Autodesk Fusion 360 part; units mm, degrees
(part 2 of 2)
sketch "Sketch3" plane through (0, 0, 0) normal (0, 0, 1) x (1, 0, 0)
  line L0 (-10.0312, 59.3426) -> (-10.0312, 45.3434)
  line L1 (-24.0307, 45.3434) -> (-24.0307, 59.3426)
  line L2 (-24.0307, 26.2934) -> (-24.0307, 40.2927)
  line L3 (-10.0312, 40.2927) -> (-10.0312, 26.2934)
  line L4 (-24.0307, 7.2434) -> (-24.0307, 21.2427)
  line L5 (-10.0312, 7.2434) -> (-24.0307, 7.2434)
  line L6 (-10.0312, 21.2427) -> (-10.0312, 7.2434)
  line L7 (-24.0307, -11.8066) -> (-24.0307, 2.1927)
  line L8 (-10.0312, -11.8066) -> (-24.0307, -11.8066)
  line L9 (-10.0312, 2.1927) -> (-10.0312, -11.8066)
  line L10 (-24.0307, -30.8568) -> (-24.0307, -16.8574)
  line L11 (-10.0312, -30.8568) -> (-24.0307, -30.8568)
  line L12 (-10.0312, -16.8574) -> (-10.0312, -30.8568)
  line L13 (-4.9807, 26.2934) -> (-4.9807, 40.2927)
  line L14 (9.0186, 26.2934) -> (-4.9807, 26.2934)
  line L15 (9.0186, 40.2927) -> (9.0186, 26.2934)
  line L16 (-4.9807, 7.2434) -> (-4.9807, 21.2427)
  line L17 (9.0186, 7.2434) -> (-4.9807, 7.2434)
  line L18 (9.0186, 21.2427) -> (9.0186, 7.2434)
  line L19 (-4.9807, -11.8066) -> (-4.9807, 2.1927)
  line L20 (9.0186, -11.8066) -> (-4.9807, -11.8066)
  line L21 (9.0186, 2.1927) -> (9.0186, -11.8066)
  line L22 (-4.9807, -30.8568) -> (-4.9807, -16.8574)
  line L23 (9.0186, -30.8568) -> (-4.9807, -30.8568)
  line L24 (9.0186, -16.8574) -> (9.0186, -30.8568)
  line L25 (14.0693, 26.2934) -> (14.0693, 40.2927)
  line L26 (28.0686, 26.2934) -> (14.0693, 26.2934)
  line L27 (14.0693, 40.2927) -> (28.0686, 40.2927)
  line L28 (14.0693, 7.2434) -> (14.0693, 21.2427)
  line L29 (28.0686, 7.2434) -> (14.0693, 7.2434)
  line L30 (28.0686, 21.2427) -> (28.0686, 7.2434)
  line L31 (14.0693, -11.8066) -> (14.0693, 2.1927)
  line L32 (28.0686, -11.8066) -> (14.0693, -11.8066)
  line L33 (28.0686, 2.1927) -> (28.0686, -11.8066)
  line L34 (14.0693, -30.8568) -> (14.0693, -16.8574)
  line L35 (28.0686, -30.8568) -> (14.0693, -30.8568)
  line L36 (28.0686, -16.8574) -> (28.0686, -30.8568)
  line L37 (33.1193, 26.2934) -> (33.1193, 40.2927)
  line L38 (47.1186, 26.2934) -> (33.1193, 26.2934)
  line L39 (47.1186, 40.2927) -> (47.1186, 26.2934)
  line L40 (33.1193, 45.3434) -> (33.1193, 59.3426)
  line L41 (39.6196, 19.9928) -> (33.3493, 19.9928)
  line L42 (32.1492, 18.2691) -> (32.1492, 14.9685)
  line L43 (32.1492, 14.9685) -> (33.3493, 14.9685)
  line L44 (33.3493, 13.2431) -> (37.8197, 13.2431)
  line L45 (33.3493, 14.9685) -> (33.3493, 13.2431)
  line L46 (33.3493, 18.2691) -> (32.1492, 18.2691)
  line L47 (33.3493, 19.9928) -> (33.3493, 18.2691)
  line L48 (37.8197, 13.2431) -> (37.8197, 11.7177)
  line L49 (37.8197, 11.7177) -> (33.1193, 11.7177)
  line L50 (42.4196, 13.2431) -> (45.6496, 13.2431)
  line L51 (47.1186, -2.2816) -> (47.1186, 11.7177)
  line L52 (47.1186, 11.7177) -> (42.4196, 11.7177)
  line L53 (42.4196, -2.2816) -> (47.1186, -2.2816)
  line L54 (33.1193, -2.2816) -> (37.8197, -2.2816)
  line L55 (33.1193, 11.7177) -> (33.1193, -2.2816)
  line L56 (37.8197, -3.8074) -> (33.3493, -3.8074)
  line L57 (32.1492, -5.5325) -> (32.1492, -8.8317)
  line L58 (33.3493, -10.5567) -> (39.6196, -10.5567)
  line L59 (45.6496, -10.5567) -> (45.6496, -3.8074)
  line L60 (42.4196, -10.5567) -> (45.6496, -10.5567)
  line L61 (45.6496, -3.8074) -> (42.4196, -3.8074)
  line L62 (39.6196, -11.3822) -> (42.4196, -11.3822)
  line L63 (42.4196, 20.8183) -> (39.6196, 20.8183)
  line L64 (45.6496, 13.2431) -> (45.6496, 19.9928)
  line L65 (45.6496, 19.9928) -> (42.4196, 19.9928)
  line L66 (42.4196, 19.9928) -> (42.4196, 20.8183)
  line L67 (39.6196, 20.8183) -> (39.6196, 19.9928)
  line L68 (42.4196, 11.7177) -> (42.4196, 13.2431)
  line L69 (37.8197, -2.2816) -> (37.8197, -3.8074)
  line L70 (42.4196, -3.8074) -> (42.4196, -2.2816)
  line L71 (33.3493, -5.5325) -> (32.1492, -5.5325)
  line L72 (33.3493, -3.8074) -> (33.3493, -5.5325)
  line L73 (32.1492, -8.8317) -> (33.3493, -8.8317)
  line L74 (33.3493, -8.8317) -> (33.3493, -10.5567)
  line L75 (39.6196, -10.5567) -> (39.6196, -11.3822)
  line L76 (42.4196, -11.3822) -> (42.4196, -10.5567)
  line L77 (14.0693, -49.9068) -> (14.0693, -35.9059)
  line L78 (28.0686, -49.9068) -> (14.0693, -49.9068)
  line L79 (28.0686, -35.9059) -> (28.0686, -49.9068)
  line L80 (33.1193, -26.3823) -> (33.1193, -40.3818)
  line L81 (47.1186, -40.3818) -> (47.1186, -26.3823)
  line L82 (45.6496, -48.6569) -> (45.6496, -41.9073)
  line L83 (45.6496, -24.8568) -> (45.6496, -18.1071)
  line L84 (47.1186, -26.3823) -> (42.4196, -26.3823)
  line L85 (37.8197, -26.3823) -> (33.1193, -26.3823)
  line L86 (33.1193, -40.3818) -> (37.8197, -40.3818)
  line L87 (42.4196, -40.3818) -> (47.1186, -40.3818)
  line L88 (45.6496, -41.9073) -> (42.4196, -41.9073)
  line L89 (37.8197, -41.9073) -> (33.3493, -41.9073)
  line L90 (33.3493, -48.6569) -> (39.6196, -48.6569)
  line L91 (39.6196, -49.4824) -> (42.4196, -49.4824)
  line L92 (42.4196, -48.6569) -> (45.6496, -48.6569)
  line L93 (32.1492, -43.6326) -> (32.1492, -46.9316)
  line L94 (33.3493, -24.8568) -> (37.8197, -24.8568)
  line L95 (42.4196, -24.8568) -> (45.6496, -24.8568)
  line L96 (45.6496, -18.1071) -> (42.4196, -18.1071)
  line L97 (39.6196, -18.1071) -> (33.3493, -18.1071)
  line L98 (42.4196, -17.2817) -> (39.6196, -17.2817)
  line L99 (32.1492, -19.8325) -> (32.1492, -23.1315)
  line L100 (42.4196, -26.3823) -> (42.4196, -24.8568)
  line L101 (37.8197, -24.8568) -> (37.8197, -26.3823)
  line L102 (32.1492, -23.1315) -> (33.3493, -23.1315)
  line L103 (33.3493, -23.1315) -> (33.3493, -24.8568)
  line L104 (33.3493, -19.8325) -> (32.1492, -19.8325)
  line L105 (33.3493, -18.1071) -> (33.3493, -19.8325)
  line L106 (39.6196, -17.2817) -> (39.6196, -18.1071)
  line L107 (42.4196, -18.1071) -> (42.4196, -17.2817)
  line L108 (37.8197, -40.3818) -> (37.8197, -41.9073)
  line L109 (42.4196, -41.9073) -> (42.4196, -40.3818)
  line L110 (32.1492, -46.9316) -> (33.3493, -46.9316)
  line L111 (33.3493, -46.9316) -> (33.3493, -48.6569)
  line L112 (33.3493, -43.6326) -> (32.1492, -43.6326)
  line L113 (33.3493, -41.9073) -> (33.3493, -43.6326)
  line L114 (39.6196, -48.6569) -> (39.6196, -49.4824)
  line L115 (42.4196, -49.4824) -> (42.4196, -48.6569)
  line L116 (-0.5063, -35.9059) -> (-14.5057, -35.9059)
  line L117 (-16.0312, -37.3762) -> (-22.7808, -37.3762)
  line L118 (-23.6063, -40.6078) -> (-23.6063, -43.4066)
  line L119 (-14.5057, -49.9068) -> (-0.5063, -49.9068)
  line L120 (-21.0555, -50.8756) -> (-17.7565, -50.8756)
  line L121 (-22.7808, -43.4066) -> (-22.7808, -49.6767)
  line L122 (-22.7808, -37.3762) -> (-22.7808, -40.6078)
  line L123 (-14.5057, -35.9059) -> (-14.5057, -40.6078)
  line L124 (-14.5057, -45.2063) -> (-14.5057, -49.9068)
  line L125 (-16.0312, -49.6767) -> (-16.0312, -45.2063)
  line L126 (7.7689, -37.3762) -> (1.0192, -37.3762)
  line L127 (7.7689, -49.6767) -> (7.7689, -43.4066)
  line L128 (7.7689, -40.6078) -> (7.7689, -37.3762)
  line L129 (1.0192, -45.2063) -> (1.0192, -49.6767)
  line L130 (2.7445, -50.8756) -> (6.0436, -50.8756)
  line L131 (-0.5063, -45.2063) -> (1.0192, -45.2063)
  line L132 (-0.5063, -49.9068) -> (-0.5063, -45.2063)
  line L133 (-17.7565, -49.6767) -> (-16.0312, -49.6767)
  line L134 (-22.7808, -49.6767) -> (-21.0555, -49.6767)
  line L135 (-16.0312, -40.6078) -> (-16.0312, -37.3762)
  line L136 (-0.5063, -40.6078) -> (-0.5063, -35.9059)
  line L137 (1.0192, -40.6078) -> (-0.5063, -40.6078)
  line L138 (1.0192, -37.3762) -> (1.0192, -40.6078)
  line L139 (8.5943, -43.4066) -> (8.5943, -40.6078)
  line L140 (8.5943, -40.6078) -> (7.7689, -40.6078)
  line L141 (7.7689, -43.4066) -> (8.5943, -43.4066)
  line L142 (1.0192, -49.6767) -> (2.7445, -49.6767)
  line L143 (2.7445, -49.6767) -> (2.7445, -50.8756)
  line L144 (6.0436, -50.8756) -> (6.0436, -49.6767)
  line L145 (6.0436, -49.6767) -> (7.7689, -49.6767)
  line L146 (-21.0555, -49.6767) -> (-21.0555, -50.8756)
  line L147 (-17.7565, -50.8756) -> (-17.7565, -49.6767)
  line L148 (-14.5057, -40.6078) -> (-16.0312, -40.6078)
  line L149 (-16.0312, -45.2063) -> (-14.5057, -45.2063)
  line L150 (-22.7808, -40.6078) -> (-23.6063, -40.6078)
  line L151 (-23.6063, -43.4066) -> (-22.7808, -43.4066)
  line L152 (-30.0717, 77.1478) -> (79.9283, 77.1478)
  line L153 (-30.0717, -55.8522) -> (-30.0717, 77.1478)
  line L154 (79.9283, -55.8522) -> (-30.0717, -55.8522)
  line L155 (79.9283, -55.8522) -> (79.9283, 77.1478)
  line L156 (0.5583, 54.6978) -> (21.2983, 54.6978)
  line L157 (21.2983, 54.6978) -> (21.2983, 64.5578)
  line L158 (0.5583, 64.5578) -> (0.5583, 54.6978)
  line L159 (86.9283, -55.8522) -> (86.9283, 77.1478)
  line L160 (-30.0717, 84.1478) -> (79.9283, 84.1478)
  line L161 (-37.0717, -55.8522) -> (-37.0717, 77.1478)
  line L162 (79.9283, -62.8522) -> (-30.0717, -62.8522)
  arc A0 (-30.0717, 84.1478) -> (-37.0717, 77.1478) centre (-30.0717, 77.1478) ccw
  arc A1 (86.9283, 77.1478) -> (79.9283, 84.1478) centre (79.9283, 77.1478) ccw
  arc A2 (79.9283, -62.8522) -> (86.9283, -55.8522) centre (79.9283, -55.8522) ccw
  arc A3 (-37.0717, -55.8522) -> (-30.0717, -62.8522) centre (-30.0717, -55.8522) ccw
  line L163 (-24.7, 58.6) -> (-11, 58.6)
  line L164 (-11, 58.6) -> (-11, 44.5)
  line L165 (-11, 44.5) -> (-24.7, 44.5)
  line L166 (-24.7, 44.5) -> (-24.7, 58.6)
  line L167 (34.1862, 59.1014) -> (48.2214, 59.1014)
  line L168 (48.2214, 59.1014) -> (48.2214, 45.0213)
  line L169 (48.2214, 45.0213) -> (34.1862, 45.0213)
  line L170 (34.1862, 45.0213) -> (34.1862, 59.1014)
  line L171 (-3, 48) -> (26, 48)
  line L172 (26, 48) -> (26, 69)
  line L173 (26, 69) -> (-3, 69)
  line L174 (-3, 69) -> (-3, 48)
  line L175 (55.1916, 78.6478) -> (79.9283, 78.6478)
  line L176 (79.9283, 78.6478) -> (79.9283, 22.183)
  line L177 (79.9283, 22.183) -> (55.1916, 22.183)
  line L178 (53.1916, 24.183) -> (53.1916, 76.6478)
  arc A4 (53.1916, 24.183) -> (55.1916, 22.183) centre (55.1916, 24.183) ccw
  arc A5 (55.1916, 78.6478) -> (53.1916, 76.6478) centre (55.1916, 76.6478) ccw
  circle A6 centre (-32.3322, 79.3113) radius 1.6
  circle A7 centre (-32.3322, -58.0158) radius 1.6
  circle A8 centre (82.1884, 79.3113) radius 1.6
  circle A9 centre (82.1884, -58.0158) radius 1.6
  circle A10 centre (-26.0717, 70.1478) radius 1.5875
  circle A11 centre (74.9283, -50.8522) radius 1.5875
  line L179 (-10.0312, 40.2927) -> (-10.0312, 26.2934)
  line L180 (-24.0307, 26.2934) -> (-24.0307, 40.2927)
  line L181 (-24.7764, 40.2927) -> (-11, 40.2927)
  line L182 (-11, 40.2927) -> (-11, 26.2934)
  line L183 (-11, 26.2934) -> (-24.7764, 26.2934)
  line L184 (-24.7764, 26.2934) -> (-24.7764, 40.2927)
  line L185 (-5.8035, 40.2927) -> (8.4714, 40.2927)
  line L186 (8.4714, 40.2927) -> (8.4714, 26.2934)
  line L187 (8.4714, 26.2934) -> (-5.8035, 26.2934)
  line L188 (-5.8035, 26.2934) -> (-5.8035, 40.2927)
  line L189 (13.5196, 40.3154) -> (27.4928, 40.3154)
  line L190 (27.4928, 40.3154) -> (27.4928, 26.2934)
  line L191 (27.4928, 26.2934) -> (13.5196, 26.2934)
  line L192 (13.5196, 26.2934) -> (13.5196, 40.3154)
  line L193 (32.4609, 40.2927) -> (46.5272, 40.2927)
  line L194 (46.5272, 40.2927) -> (46.5272, 26.2934)
  line L195 (46.5272, 26.2934) -> (32.4609, 26.2934)
  line L196 (32.4609, 26.2934) -> (32.4609, 40.2927)
  line L197 (13.3868, 21.2427) -> (27.44, 21.2427)
  line L198 (27.44, 21.2427) -> (27.44, 7.2434)
  line L199 (27.44, 7.2434) -> (13.3868, 7.2434)
  line L200 (13.3868, 7.2434) -> (13.3868, 21.2427)
  line L201 (-6.0185, 21.2427) -> (8, 21.2427)
  line L202 (8, 21.2427) -> (8, 7.2434)
  line L203 (8, 7.2434) -> (-6.0185, 7.2434)
  line L204 (-6.0185, 7.2434) -> (-6.0185, 21.2427)
  line L205 (-24.847, 21.2427) -> (-11, 21.2427)
  line L206 (-11, 21.2427) -> (-11, 7.2434)
  line L207 (-11, 7.2434) -> (-24.847, 7.2434)
  line L208 (-24.847, 7.2434) -> (-24.847, 21.2427)
  line L209 (-24.847, 2.1927) -> (-11, 2.1927)
  line L210 (-11, 2.1927) -> (-11, -11.8066)
  line L211 (-11, -11.8066) -> (-24.847, -11.8066)
  line L212 (-24.847, -11.8066) -> (-24.847, 2.1927)
  line L213 (-5.6672, 2.1927) -> (7.7516, 2.1927)
  line L214 (7.7516, 2.1927) -> (7.7516, -11.8066)
  line L215 (7.7516, -11.8066) -> (-5.6672, -11.8066)
  line L216 (-5.6672, -11.8066) -> (-5.6672, 2.1927)
  line L217 (13.1612, 2.1927) -> (27, 2.1927)
  line L218 (27, 2.1927) -> (27, -11.8066)
  line L219 (27, -11.8066) -> (13.1612, -11.8066)
  line L220 (13.1612, -11.8066) -> (13.1612, 2.1927)
  line L221 (13.1612, -16.8574) -> (27, -16.8574)
  line L222 (27, -16.8574) -> (27, -30.8568)
  line L223 (27, -30.8568) -> (13.1612, -30.8568)
  line L224 (13.1612, -30.8568) -> (13.1612, -16.8574)
  line L225 (-6.2995, -16.8574) -> (8, -16.8574)
  line L226 (8, -16.8574) -> (8, -30.8568)
  line L227 (8, -30.8568) -> (-6.2995, -30.8568)
  line L228 (-6.2995, -30.8568) -> (-6.2995, -16.8574)
  line L229 (-25.2685, -16.8574) -> (-11, -16.8574)
  line L230 (-11, -16.8574) -> (-11, -30.8568)
  line L231 (-11, -30.8568) -> (-25.2685, -30.8568)
  line L232 (-25.2685, -30.8568) -> (-25.2685, -16.8574)
  line L233 (13, -36) -> (27.0093, -35.9059)
  line L234 (27.0093, -35.9059) -> (27.1032, -49.9062)
  line L235 (27.1032, -49.9062) -> (13.094, -50.0002)
  line L236 (13.094, -50.0002) -> (13, -36)
  point P0 (33.1193, 26.2934)
  point P1 (42.4196, 11.7177)
  point P2 (33.3493, -8.8317)
  point P3 (45.6496, -48.6569)
  point P4 (32.1492, -19.8325)
  dimension "d2" = 7
  dimension "d3" = 2
  dimension "d4" = 3.2
  constraint tangent L160 A0
  constraint tangent L161 A0
  constraint tangent L159 A1
  constraint tangent L160 A1
  constraint equal A0 A1
  constraint tangent L159 A2
  constraint tangent L162 A2
  constraint equal A0 A2
  constraint tangent L161 A3
  constraint tangent L162 A3
  constraint equal A0 A3
  constraint horizontal L163
  constraint vertical L164
  constraint horizontal L165
  constraint vertical L166
  constraint horizontal L167
  constraint vertical L168
  constraint horizontal L169
  constraint vertical L170
  constraint horizontal L171
  constraint vertical L172
  constraint horizontal L173
  constraint vertical L174
  constraint horizontal L175
  constraint vertical L176
  constraint horizontal L177
  constraint vertical L178
  constraint coincident L155 L176.end
  constraint tangent L177 A4
  constraint tangent L178 A4
  constraint tangent L175 A5
  constraint tangent L178 A5
  constraint equal A4 A5
  constraint vertical L179
  constraint vertical L180
  constraint coincident L3.end L179.end
  constraint coincident L2.end L180.end
  constraint perpendicular L181 L182
  constraint parallel L181 L183
  constraint parallel L182 L184
  constraint perpendicular L179 L181
  constraint perpendicular L185 L186
  constraint parallel L185 L187
  constraint parallel L186 L188
  constraint perpendicular L15 L185
  constraint horizontal L189
  constraint vertical L190
  constraint horizontal L191
  constraint vertical L192
  constraint coincident L26 L190.end
  constraint perpendicular L193 L194
  constraint parallel L193 L195
  constraint parallel L194 L196
  constraint perpendicular L39 L193
  constraint perpendicular L197 L198
  constraint parallel L197 L199
  constraint parallel L198 L200
  constraint perpendicular L30 L197
  constraint perpendicular L201 L202
  constraint parallel L201 L203
  constraint parallel L202 L204
  constraint perpendicular L18 L201
  constraint perpendicular L205 L206
  constraint parallel L205 L207
  constraint parallel L206 L208
  constraint perpendicular L4 L205
  constraint perpendicular L209 L210
  constraint parallel L209 L211
  constraint parallel L210 L212
  constraint perpendicular L7 L209
  constraint perpendicular L213 L214
  constraint parallel L213 L215
  constraint parallel L214 L216
  constraint perpendicular L19 L213
  constraint perpendicular L217 L218
  constraint parallel L217 L219
  constraint parallel L218 L220
  constraint perpendicular L33 L217
  constraint perpendicular L221 L222
  constraint parallel L221 L223
  constraint parallel L222 L224
  constraint perpendicular L34 L221
  constraint perpendicular L225 L226
  constraint parallel L225 L227
  constraint parallel L226 L228
  constraint perpendicular L22 L225
  constraint perpendicular L229 L230
  constraint parallel L229 L231
  constraint parallel L230 L232
  constraint perpendicular L10 L229
  constraint perpendicular L233 L234
  constraint parallel L233 L235
  constraint parallel L234 L236
  measures "d2" radius of A0
  measures "d3" radius of A4
  measures "d4" diameter of A6
extrude "Extrude1" add sketch "Sketch3" along normal blind 3 contours L2 L180 L181 L183 L184 | L2 L180 L181 L182 L183 | L4 L205 L207 L208 | L4 L5 L205 L206 L207 | L7 L209 L211 L212 | L7 L8 L209 L210 L211 | L10 L229 L231 L232 | L10 L11 L229 L230 L231 | L13 L185 L187 L188 | L13 L14 L185 L186 L187 | L16 L201 L203 L204 | L16 L17 L201 L202 L203 | L19 L213 L215 L216 | L19 L20 L213 L214 L215 | L22 L225 L227 L228 | L22 L23 L225 L226 L227 | L25 L27 L189 L190 L191 L192 | L25 L26 L27 L190 L191 | L28 L197 L199 L200 | L28 L29 L197 L198 L199 | L31 L217 L219 L220 | L31 L32 L217 L218 L219 | L34 L221 L223 L224 | L34 L35 L221 L222 L223 | L37 L193 L195 L196 | L37 L38 L193 L194 L195 | L77 L78 L233 L235 L236 | L77 L78 L233 L234 | L152 L153 L154 L155 L177 L178 A4 A5 | L159 L160 L161 L162 A0 A1 A2 A3 | A10 | A11 makes body 1
delete_body "RemoveBody1" bodies 1
extrude "Extrude2" add sketch "Sketch3" along normal blind 3 separate body contours L4 L205 L207 L208 | L4 L5 L205 L206 L207 | L7 L209 L211 L212 | L7 L8 L209 L210 L211 | L10 L229 L231 L232 | L10 L11 L229 L230 L231 | L13 L185 L187 L188 | L13 L14 L185 L186 L187 | L16 L201 L203 L204 | L16 L17 L201 L202 L203 | L19 L213 L215 L216 | L19 L20 L213 L214 L215 | L22 L225 L227 L228 | L22 L23 L225 L226 L227 | L25 L27 L189 L190 L191 L192 | L25 L26 L27 L190 L191 | L28 L197 L199 L200 | L28 L29 L197 L198 L199 | L31 L217 L219 L220 | L31 L32 L217 L218 L219 | L34 L221 L223 L224 | L34 L35 L221 L222 L223 | L37 L193 L195 L196 | L37 L38 L193 L194 L195 | L77 L78 L233 L235 L236 | L77 L78 L233 L234 | L152 L153 L154 L155 L177 L178 A4 A5 | L159 L160 L161 L162 A0 A1 A2 A3 | A10 | A11 makes body 2
delete_body "RemoveBody2" bodies 2
extrude "Extrude3" add sketch "Sketch3" along normal blind 3 separate body contours L152 L153 L154 L155 L177 L178 A4 A5 | L159 L160 L161 L162 A0 A1 A2 A3 | A10 | A11 makes body 3
sketch "pico_usb_opening" plane through (0, 84.1478, 0) normal (0, 1, 0) x (-1, 0, 0)
  line L0 (-76.9201, -8.4888) -> (30.0799, -8.4888)
  line L1 (30.0799, 0.0112) -> (-76.9201, 0.0112)
  line L2 (30.0799, -8.4888) -> (30.0799, 0.0112)
  line L3 (-76.9201, 0.0112) -> (-76.9201, -8.4888)
  spline S0 degree 3 poles (-62.4158, 2.0177) (-62.362, 2.0707) (-62.3197, 2.1361) (-62.2937, 2.2023) (-62.2678, 2.2685) (-62.2577, 2.3357) (-62.2577, 2.3932) knots 0 0 0 0 0.000228 0.000228 0.000228 0.000456 0.000456 0.000456 0.000456
  line L4 (-63.5977, 1.2561) -> (-63.5977, 1.5361)
  line L5 (-62.4229, 2.0108) -> (-63.0194, 1.4143)
  arc A0 (-63.4012, 1.5361) -> (-63.2174, 1.6123) centre (-63.4012, 1.7961) ccw
  line L6 (-63.4012, 1.2561) -> (-63.5977, 1.2561)
  arc A1 (-63.0194, 1.4143) -> (-63.4012, 1.2561) centre (-63.4012, 1.7961) cw
  line L7 (-63.5977, 1.5361) -> (-63.4012, 1.5361)
  line L8 (-62.8189, 2.0108) -> (-62.4229, 2.0108)
  line L9 (-63.2174, 1.6123) -> (-62.8189, 2.0108)
  line L10 (-69.5724, 2.0108) -> (-68.9759, 1.4143)
  line L11 (-68.5941, 1.2561) -> (-68.3977, 1.2561)
  arc A2 (-68.9759, 1.4143) -> (-68.5941, 1.2561) centre (-68.5941, 1.7961) ccw
  line L12 (-69.1764, 2.0108) -> (-69.5724, 2.0108)
  line L13 (-68.778, 1.6123) -> (-69.1764, 2.0108)
  line L14 (-68.3977, 1.5361) -> (-68.5941, 1.5361)
  line L15 (-68.3977, 1.2561) -> (-68.3977, 1.5361)
  arc A3 (-68.5941, 1.5361) -> (-68.778, 1.6123) centre (-68.5941, 1.7961) cw
  line L16 (-69.5724, 2.0108) -> (-69.1764, 2.0108)
  spline S1 degree 3 poles (-69.3815, 2.2124) (-69.3817, 2.2126) (-69.3819, 2.2128) (-69.3894, 2.2209) (-69.396, 2.2289) (-69.4172, 2.2577) (-69.4289, 2.2793) (-69.4378, 2.302) (-69.4381, 2.3026) (-69.4385, 2.3035) (-69.4386, 2.3038) (-69.4387, 2.3043) (-69.4388, 2.3044) (-69.4389, 2.3047) (-69.4389, 2.3048) (-69.439, 2.3049) (-69.439, 2.3049) (-69.439, 2.305) (-69.439, 2.305) (-69.4416, 2.3117) (-69.4444, 2.3201) (-69.452, 2.3472) (-69.4549, 2.3641) (-69.457, 2.3844) (-69.4573, 2.3883) (-69.4576, 2.3928) (-69.4576, 2.3929) (-69.4577, 2.3932) knots -0.000094 -0.000094 -0.000094 -0.000094 0 0 0.003326 0.003326 0.01148 0.01148 0.011712 0.011712 0.011827 0.011827 0.011884 0.011884 0.011913 0.011913 0.011927 0.011927 0.011941 0.011941 0.01441 0.01441 0.018676 0.018676 0.019737 0.019737 0.019799 0.019799 0.019799 0.019799
  line L17 (-69.4577, 2.3932) -> (-69.4577, 2.5961)
  line L18 (-69.4577, 2.5961) -> (-69.7377, 2.5961)
  line L19 (-69.7377, 2.5961) -> (-69.7377, 2.3932)
  ellipse E0 centre (-69.5176, 2.3374) end of major axis (-69.456, 2.0035) minor radius 0.2149 (-69.7377, 2.3932) -> (-69.7015, 2.2021) ccw
  ellipse E1 centre (-69.4321, 2.2443) end of major axis (-69.2216, 1.9336) minor radius 0.2595 (-69.7015, 2.2021) -> (-69.5795, 2.0177) ccw
  line L20 (-67.7634, 3.3184) -> (-67.9685, 3.1133)
  line L21 (-69.3744, 2.2229) -> (-69.2623, 2.1108)
  line L22 (-69.4674, 1.9057) -> (-69.5795, 2.0179)
  arc A4 (-68.3756, 3.6861) -> (-67.9584, 3.5133) centre (-68.3756, 3.0961) cw
  arc A5 (-69.5795, 2.0179) -> (-69.7377, 2.3997) centre (-69.1977, 2.3997) cw
  arc A6 (-69.4477, 2.3997) -> (-69.3744, 2.2229) centre (-69.1977, 2.3997) ccw
  line L23 (-69.1977, 3.6861) -> (-68.3756, 3.6861)
  line L24 (-67.9685, 3.1133) -> (-68.1635, 3.3083)
  line L25 (-69.7377, 2.3997) -> (-69.7377, 3.1461)
  line L26 (-68.3756, 3.3961) -> (-69.1977, 3.3961)
  arc A7 (-69.1977, 3.3961) -> (-69.4477, 3.1461) centre (-69.1977, 3.1461) ccw
  arc A8 (-68.1635, 3.3083) -> (-68.3756, 3.3961) centre (-68.3756, 3.0961) ccw
  arc A9 (-69.7377, 3.1461) -> (-69.1977, 3.6861) centre (-69.1977, 3.1461) cw
  line L27 (-69.4477, 3.1461) -> (-69.4477, 2.3997)
  line L28 (-67.9584, 3.5133) -> (-67.7634, 3.3184)
  line L29 (-69.2623, 2.1108) -> (-69.4674, 1.9057)
  line L30 (-64.2319, 3.3184) -> (-64.0268, 3.1133)
  line L31 (-62.2577, 2.3997) -> (-62.2577, 3.1461)
  line L32 (-62.7977, 3.6861) -> (-63.6197, 3.6861)
  line L33 (-64.0268, 3.1133) -> (-63.8319, 3.3083)
  arc A10 (-63.8319, 3.3083) -> (-63.6197, 3.3961) centre (-63.6197, 3.0961) cw
  line L34 (-64.0369, 3.5133) -> (-64.2319, 3.3184)
  line L35 (-63.6197, 3.3961) -> (-62.7977, 3.3961)
  line L36 (-62.5477, 3.1461) -> (-62.5477, 2.3997)
  arc A11 (-62.5477, 2.3997) -> (-62.6209, 2.2229) centre (-62.7977, 2.3997) cw
  line L37 (-62.6209, 2.2229) -> (-62.733, 2.1108)
  arc A12 (-62.7977, 3.3961) -> (-62.5477, 3.1461) centre (-62.7977, 3.1461) cw
  line L38 (-62.733, 2.1108) -> (-62.528, 1.9057)
  arc A13 (-62.4158, 2.0179) -> (-62.2577, 2.3997) centre (-62.7977, 2.3997) ccw
  line L39 (-62.528, 1.9057) -> (-62.4158, 2.0179)
  arc A14 (-62.2577, 3.1461) -> (-62.7977, 3.6861) centre (-62.7977, 3.1461) ccw
  arc A15 (-63.6197, 3.6861) -> (-64.0369, 3.5133) centre (-63.6197, 3.0961) ccw
  line L40 (-63.614, 3.6861) -> (-63.614, 3.3961)
  line L41 (-64.7977, 3.3961) -> (-64.7977, 3.6861)
  line L42 (-63.614, 3.3961) -> (-64.7977, 3.3961)
  line L43 (-64.7977, 3.6861) -> (-63.614, 3.6861)
  line L44 (-64.8077, 3.3961) -> (-67.1877, 3.3961)
  line L45 (-67.1877, 3.6961) -> (-64.8077, 3.6961)
  line L46 (-64.8077, 3.6961) -> (-64.8077, 3.3961)
  line L47 (-67.1877, 3.3961) -> (-67.1877, 3.6961)
  line L48 (-67.1977, 3.6861) -> (-67.1977, 3.3961)
  line L49 (-68.3813, 3.6861) -> (-67.1977, 3.6861)
  line L50 (-67.1977, 3.3961) -> (-68.3813, 3.3961)
  line L51 (-68.3813, 3.3961) -> (-68.3813, 3.6861)
sketch "Sketch5" plane through (0, 84.1478, 0) normal (0, 1, 0) x (-1, 0, 0)
  line L0 (-79.9283, 0) -> (30.0717, 0)
  line L1 (30.0717, 0) -> (30.0717, 3)
  line L2 (30.0717, 3) -> (-79.9283, 3)
  line L3 (-79.9283, 3) -> (-79.9283, 0)
  line L4 (-69.75, 3) -> (-62.25, 3)
  line L5 (-62.25, 3) -> (-62.25, 2.2)
  line L6 (-63.25, 1.2) -> (-68.75, 1.2)
  line L7 (-69.75, 2.2) -> (-69.75, 3)
  arc A0 (-63.25, 1.2) -> (-62.25, 2.2) centre (-63.25, 2.2) ccw
  arc A1 (-69.75, 2.2) -> (-68.75, 1.2) centre (-68.75, 2.2) ccw
  line L8 (-62.2577, 2.3997) -> (-62.2577, 3.1461)
  arc A2 (-62.2577, 3.1461) -> (-62.7977, 3.6861) centre (-62.7977, 3.1461) ccw
  line L9 (-62.7977, 3.6861) -> (-63.6197, 3.6861)
  line L10 (-64.7977, 3.6861) -> (-63.614, 3.6861)
  line L11 (-67.1877, 3.6961) -> (-64.8077, 3.6961)
  line L12 (-68.3813, 3.6861) -> (-67.1977, 3.6861)
  arc A3 (-69.1977, 3.6861) -> (-69.7377, 3.1461) centre (-69.1977, 3.1461) ccw
  line L13 (-69.1977, 3.6861) -> (-68.3756, 3.6861)
  dimension "d11" = 1
  constraint perpendicular L4 L5
  constraint parallel L4 L6
  constraint parallel L5 L7
  constraint coincident L2 L4.end
  constraint coincident L2 L4.start
  constraint tangent L5 A0
  constraint tangent L6 A0
  constraint tangent L6 A1
  constraint tangent L7 A1
  constraint equal A0 A1
  measures "d11" radius of A0
extrude "Extrude4" cut sketch "Sketch5" against normal blind 10 contours L2 L4 L5 L6 L7 A0 A1 bodies 3
extrude "Extrude5" cut sketch "Sketch5" against normal blind 44.5 contours L2 L4 L5 L6 L7 A0 A1 bodies 3
